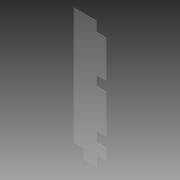
# Autodesk Inventor part: tower walls
Saved by Autodesk Inventor 2011 SP1 (Build 150282100, 282)
## iProperties
Created: 2012-01-20
Part Number: tower walls
Document SubType Name: Modeling
Designer: Christopher
Density: 1 g/cm^3
Author: Christopher
Autodesk Inventor part; units mm, degrees
ref_plane "YZ Plane" through (0, 0, 0) normal (1, 0, 0) x (0, 1, 0)
ref_plane "XZ Plane" through (0, 0, 0) normal (0, 1, 0) x (-1, 0, 0)
ref_plane "XY Plane" through (0, 0, 0) normal (0, 0, 1) x (1, 0, 0)
sketch "Sketch1" plane through (0, 0, 0) normal (0, 0, 1) x (1, 0, 0)
  line L0 (176.5882, -640.9214) -> (176.5882, 349.6786)
  line L1 (176.5882, 349.6786) -> (-77.4118, 349.6786)
  line L2 (-77.4118, 349.6786) -> (-77.4118, -640.9214)
  line L3 (100.3882, -640.9214) -> (100.3882, -564.7214)
  line L4 (100.3882, -564.7214) -> (176.5882, -564.7214)
  line L5 (176.5882, -475.8214) -> (100.3882, -475.8214)
  line L6 (100.3882, -475.8214) -> (100.3882, -399.6214)
  line L7 (100.3882, -399.6214) -> (176.5882, -399.6214)
  line L8 (176.5882, -399.6214) -> (176.5882, -475.8214)
  line L9 (176.5882, -94.8214) -> (100.3882, -94.8214)
  line L10 (100.3882, -94.8214) -> (100.3882, 70.2786)
  line L11 (100.3882, 70.2786) -> (176.5882, 70.2786)
  line L12 (176.5882, 70.2786) -> (176.5882, -94.8214)
  line L13 (176.5882, 349.6786) -> (100.3882, 349.6786)
  line L14 (100.3882, 349.6786) -> (100.3882, 273.4786)
  line L15 (100.3882, 273.4786) -> (176.5882, 273.4786)
  line L16 (176.5882, 273.4786) -> (176.5882, 349.6786)
  line L17 (-77.4118, 275.381) -> (-77.4118, 369.0362)
  line L18 (-77.4118, -16.7496) -> (-77.4118, 88.2844)
  line L19 (-77.4118, -379.8866) -> (-77.4118, -294.668)
  line L20 (-77.4118, -640.9214) -> (-1.2118, -640.9214)
  line L21 (-1.2118, -640.9214) -> (-1.2118, -564.7214)
  line L22 (-1.2118, -564.7214) -> (-77.4118, -564.7214)
  line L23 (-77.4118, -564.7214) -> (-77.4118, -640.9214)
  line L24 (-77.4118, -259.9214) -> (-1.2118, -259.9214)
  line L25 (-1.2118, -259.9214) -> (-1.2118, -336.1214)
  line L26 (-1.2118, -336.1214) -> (-77.4118, -336.1214)
  line L27 (-77.4118, -336.1214) -> (-77.4118, -259.9214)
  line L28 (-77.4118, -5.9214) -> (-1.2118, -5.9214)
  line L29 (-1.2118, -5.9214) -> (-1.2118, 70.2786)
  line L30 (-1.2118, 70.2786) -> (-77.4118, 70.2786)
  line L31 (-77.4118, 70.2786) -> (-77.4118, -5.9214)
  line L32 (-77.4118, 349.6786) -> (-1.2118, 349.6786)
  line L33 (-1.2118, 349.6786) -> (-1.2118, 273.4786)
  line L34 (-1.2118, 273.4786) -> (-77.4118, 273.4786)
  line L35 (-77.4118, 273.4786) -> (-77.4118, 349.6786)
  line L36 (100.3882, -640.9214) -> (100.3882, -666.3214)
  line L37 (100.3882, -666.3214) -> (-1.2118, -666.3214)
  line L38 (-1.2118, -666.3214) -> (-1.2118, -640.9214)
  point P0 (0, 0)
  point P1 (49.5882, -323.4214)
  point P2 (-64.7118, -437.7214)
  point P3 (-64.7118, -132.9214)
  point P4 (163.8882, 171.8786)
  point P5 (-64.7118, 171.8786)
  point P6 (163.8882, -196.4214)
  point P7 (163.8882, -513.9214)
  point P8 (49.5882, -653.6214)
  point P9 (49.5882, 6.7786)
  dimension "d0" = 254
  dimension "d1" = 990.6
  dimension "d2" = 76.2
  dimension "d3" = 76.2
  dimension "d4" = 76.2
  dimension "d5" = 76.2
  dimension "d6" = 88.9
  dimension "d7" = 304.8
  dimension "d8" = 203.2
  dimension "d9" = 76.2
  dimension "d10" = 76.2
  dimension "d11" = 76.2
  dimension "d14" = 76.2
  dimension "d15" = 76.2
  dimension "d16" = 76.2
  dimension "d17" = 76.2
  dimension "d18" = 63.5
  dimension "d19" = 76.2
  dimension "d20" = 76.2
  dimension "d21" = 203.2
  dimension "d22" = 76.2
  dimension "d23" = 76.2
  dimension "d24" = 12.7
  dimension "d25" = 12.7
  dimension "d26" = 101.6
  dimension "d27" = 101.6
  dimension "d28" = 127
  dimension "d29" = 12.7
  dimension "d30" = 12.7
  dimension "d31" = 127
  dimension "d32" = 101.6
  dimension "d33" = 12.7
  dimension "d34" = 12.7
  dimension "d35" = 101.6
  dimension "d36" = 38.1
  dimension "d37" = 25.4
  dimension "d38" = 101.6
  dimension "d46" = 12.7
  constraints: 78 end point, 18 parallel, 9 perpendicular, 8 point on line, 7 horizontal
  measures "d0" distance of L0.end L1.end
  measures "d1" distance of L1.end L2.end
  measures "d2" distance of L3.start L3.end
  measures "d3" distance of L3.end L4.end
  measures "d4" distance of L5.end L6.end
  measures "d5" distance of L6.end L7.end
  measures "d6" distance between parallel lines of L5 L4
  measures "d7" distance between parallel lines of L9 L7
  measures "d8" distance between parallel lines of L11 L15
  measures "d9" distance of L13.end L14.end
  measures "d10" distance of L10.end L11.end
  measures "d11" distance of L14.end L15.end
  measures "d14" distance of L21.end L22.end
  measures "d15" distance of L20.end L21.end
  measures "d16" distance of L24.start L24.end
  measures "d17" distance of L24.end L25.end
  measures "d18" distance between parallel lines of L7 L26
  measures "d19" distance of L28.end L29.end
  measures "d20" distance of L29.end L30.end
  measures "d21" distance between parallel lines of L15 L30
  measures "d22" distance of L32.end L33.end
  measures "d23" distance of L33.end L34.end
  measures "d24" distance from line of L2 point (-64.712, 171.879)
  measures "d25" distance from line of L0 point (163.888, 171.879)
  measures "d26" distance from line of L34 point (-64.712, 171.879)
  measures "d27" distance from line of L15 point (163.888, 171.879)
  measures "d28" distance from line of L28 point (-64.712, -132.921)
  measures "d29" distance from line of L2 point (-64.712, -132.921)
  measures "d30" distance from line of L26 point (49.588, -323.421)
  measures "d31" distance from line of L0 point (49.588, -323.421)
  measures "d32" distance from line of L26 point (-64.712, -437.721)
  measures "d33" distance from line of L2 point (-64.712, -437.721)
  measures "d34" distance from line of L0 point (163.888, -196.421)
  measures "d35" distance from line of L9 point (163.888, -196.421)
  measures "d36" distance from line of L5 point (163.888, -513.921)
  measures "d37" distance of L3.start L36.end
  measures "d38" distance of L36.end L37.end
  measures "d46" distance from line of L28 point (49.588, 6.779)
extrude "Extrusion1" add sketch "Sketch1" against normal blind 3.175 contours L4 L3 L36 L37 L38 L21 L22 L2 L26 L25 L24 L28 L29 L30 L34 L33 L1 L14 L15 L0 L11 L10 L9 L7 L6 L5
hole "Hole1" at (49.5882, -323.4214, 0) at (-64.7118, -437.7214, 0) at (-64.7118, -132.9214, 0) at (163.8882, 171.8786, 0) at (-64.7118, 171.8786, 0) at (163.8882, -196.4214, 0) at (163.8882, -513.9214, 0) at (49.5882, -653.6214, 0) at (49.5882, 6.7786, 0) direction (0, 0, -1) diameter 6.35 depth 25.4 tip angle 118
body "Solid1"
